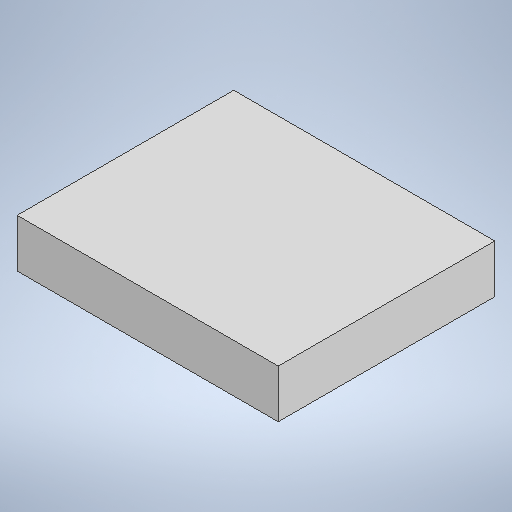
# Autodesk Inventor part: Hardware_container-lid
Saved by Autodesk Inventor 2025.1 (Build 291241000, 241)
## iProperties
Created: 2025-05-21
Part Number: Hardware_container-lid
Material: Générique
Document SubType Name: Modeling
Designer: ewenm
Density: 1 g/cm^3
Appearance: Par défaut
Author: ewenm
Autodesk Inventor part; units mm, degrees
ref_plane "YZ Plane" through (0, 0, 0) normal (1, 0, 0) x (0, 1, 0)
ref_plane "XZ Plane" through (0, 0, 0) normal (0, 1, 0) x (-1, 0, 0)
ref_plane "XY Plane" through (0, 0, 0) normal (0, 0, 1) x (1, 0, 0)
sketch "Esquisse1" plane through (0, 0, 0) normal (0, 1, 0) x (-1, 0, 0)
  line L0 (0, -72.9333) -> (0, 73.0667)
  line L1 (88, 0.0667) -> (-88, 0.0667)
  line L2 (88, -72.9333) -> (-88, -72.9333)
  line L3 (-88, -72.9333) -> (-88, 73.0667)
  line L4 (-88, 73.0667) -> (88, 73.0667)
  line L5 (88, 73.0667) -> (88, -72.9333)
  point P0 (0, 0)
  dimension "d0" = 176
  dimension "d1" = 146
  constraints: 12 end point, 4 midpoint, 2 horizontal, 2 parallel, 1 perpendicular, 1 vertical, 2 other
  measures "d0" distance between parallel lines of L3 L5
  measures "d1" distance between parallel lines of L4 L2
extrude "Extrusion1" add sketch "Esquisse1" along normal blind 2
sketch "Esquisse3" plane through (0, 0, 0) normal (0, -1, 0) x (1, 0, 0)
  line L0 (-83, 68.0667) -> (83, 68.0667)
  line L1 (83, 68.0667) -> (83, -67.9333)
  line L2 (83, -67.9333) -> (-83, -67.9333)
  line L3 (-83, -67.9333) -> (-83, 68.0667)
  line L4 (-88, 73.0667) -> (88, 73.0667) projected
  line L5 (88, 73.0667) -> (88, -72.9333) projected
  line L6 (88, -72.9333) -> (-88, -72.9333) projected
  line L7 (-88, -72.9333) -> (-88, 73.0667) projected
  point P0 (0, 0)
  dimension "d4" = 5
  dimension "d5" = 5
  dimension "d6" = 5
  dimension "d7" = 5
  constraints: 8 end point, 2 parallel, 1 horizontal, 1 perpendicular
  measures "d4" distance between parallel lines of L4 L0
  measures "d5" distance between parallel lines of L5 L1
  measures "d6" distance between parallel lines of L6 L2
  measures "d7" distance between parallel lines of L7 L3
extrude "Extrusion2" add sketch "Esquisse3" along normal blind 24.5
sketch "Esquisse4" plane through (0, -24.5, 0) normal (0, -1, 0) x (1, 0, 0)
  line L0 (-86.5, 71.5667) -> (86.5, 71.5667)
  line L1 (86.5, 71.5667) -> (86.5, -71.4333)
  line L2 (86.5, -71.4333) -> (-86.5, -71.4333)
  line L3 (-86.5, -71.4333) -> (-86.5, 71.5667)
  line L4 (88, 73.0667) -> (-88, 73.0667) projected
  line L5 (88, -72.9333) -> (88, 73.0667) projected
  line L6 (-88, -72.9333) -> (88, -72.9333) projected
  line L7 (-88, 73.0667) -> (-88, -72.9333) projected
  point P0 (0, 0)
  dimension "d10" = 1.5
  dimension "d11" = 1.5
  dimension "d12" = 1.5
  dimension "d13" = 1.5
  constraints: 8 end point, 2 parallel, 1 horizontal, 1 perpendicular
  measures "d10" distance between parallel lines of L0 L4
  measures "d11" distance between parallel lines of L5 L1
  measures "d12" distance between parallel lines of L6 L2
  measures "d13" distance between parallel lines of L3 L7
extrude "Extrusion3" add sketch "Esquisse4" along normal blind 6
